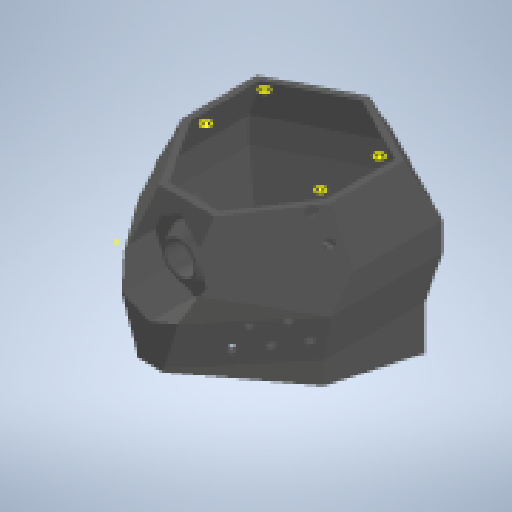
# Autodesk Inventor part: head_bace
Saved by Autodesk Inventor 2026.1 (Build 301233020, 233B)
## iProperties
Created: 2024-02-25
Part Number: head_bace
Material: 一般
Document SubType Name: Modeling
Designer: hibik
Density: 1 g/cm^3
Appearance: 既定
Author: hibik
Autodesk Inventor part; units mm, degrees
ref_plane "YZ Plane" through (0, 0, 0) normal (1, 0, 0) x (0, 1, 0)
ref_plane "XZ Plane" through (0, 0, 0) normal (0, 1, 0) x (-1, 0, 0)
sketch "スケッチ1" plane through (0, 0, 0) normal (0, 1, 0) x (-1, 0, 0)
  line L0 (-17.5, -21) -> (0, 0)
  line L1 (0, 0) -> (17.5, -21)
  line L2 (17.5, -21) -> (17.5, -41)
  line L3 (17.5, -41) -> (0, -50)
  line L4 (0, -50) -> (-17.5, -41)
  line L5 (-17.5, -41) -> (-17.5, -21)
  line L6 (0, -60) -> (0, 10) projected
  line L7 (24.5, 0) -> (-24.5, 0) projected
  dimension "d0" = 50
  dimension "d12" = 35
  dimension "d13" = 20
  dimension "d14" = 21
  constraints: 12 end point, 2 horizontal alignment, 1 coincident, 1 point on line, 1 vertical, 2 other
  measures "d0" distance of L0.end L3.end
  measures "d12" distance between parallel lines of L5 L2
  measures "d13" distance of L4.end L0.start
  measures "d14" vertical distance of L0.end L1.end
extrude "押し出し1" add sketch "スケッチ1" along normal blind 18
chamfer "面取り1" distance 5 distance2 10 6 edges at (8.75, 18, -10.5) (17.5, 18, -31) (8.75, 18, -45.5) (-8.75, 18, -45.5) (-17.5, 18, -31) (-8.75, 18, -10.5) measured on face at (8.3659, 18, -10.8201) measured on face at (-8.3659, 18, -10.8201) measured on face at (8.5213, 18, -45.0554) measured on face at (17, 18, -31) measured on face at (-17, 18, -31) measured on face at (-8.5213, 18, -45.0554)
extrude "押し出し2" add sketch "スケッチ1" against normal blind 5
ref_plane "作業平面1" through (0, 8, 0) normal (0, -0.7881104, 0.6155339) x (1, 0, 0)
sketch "スケッチ2" plane through (0, 8, 0) normal (0, -0.7881104, 0.6155339) x (1, 0, 0)
  line L0 (0, 0) -> (17.5, -16.5503) projected
  line L1 (-17.5, -16.5503) -> (0, 0) projected
  line L2 (-5, -4.7287) -> (-5, -4.7287)
  line L3 (-5, -4.7287) -> (5, -4.7287)
  line L4 (13.3346, -12.611) -> (5, -4.7287)
  line L5 (-5, -4.7287) -> (-23.6413, -26.9446)
  line L6 (5, -4.7287) -> (18.7173, -21.0763)
  line L7 (-23.6413, -26.9446) -> (-26.2109, -24.7885)
  line L8 (-26.2109, -24.7885) -> (-17.5, -16.5503)
  line L9 (17.5, -16.5503) -> (23.8178, -21.8516)
  line L10 (23.8178, -21.8516) -> (18.7173, -21.0763)
  point P0 (0, -4.9243)
  dimension "d9" = 10
  dimension "d25" = 130
  dimension "d26" = 130
  constraints: 18 end point, 4 point on line, 2 collinear, 1 horizontal, 1 parallel
  measures "d9" distance of L2.end L3.end
  measures "d25" angle of L3 L5
  measures "d26" angle of L6 L3
extrude "押し出し3" cut sketch "スケッチ2" against normal through all
chamfer "面取り2" distance 2 distance2 8 6 edges at (-8.75, -5, -10.5) (-17.5, -5, -31) (-8.75, -5, -45.5) (8.75, -5, -45.5) (17.5, -5, -31) (8.75, -5, -10.5) measured on face at (17, -5, -31) measured on face at (-8.5213, -5, -45.0554) measured on face at (8.3659, -5, -10.8201) measured on face at (-17, -5, -31) measured on face at (-8.3659, -5, -10.8201) measured on face at (8.5213, -5, -45.0554)
sketch "スケッチ3" plane through (0, -5, 0) normal (0, -1, 0) x (1, 0, 0)
  line L0 (0, -3.1241) -> (15.5, -21.7241) projected
  line L1 (-15.5, -21.7241) -> (0, -3.1241) projected
  line L2 (-15.5, -39.7796) -> (-15.5, -21.7241) projected
  line L3 (0, -47.751) -> (-15.5, -39.7796) projected
  line L4 (15.5, -39.7796) -> (0, -47.751) projected
  line L5 (15.5, -21.7241) -> (15.5, -39.7796) projected
  point P0 (0, 0)
extrude "押し出し4" add sketch "スケッチ3" along normal blind 8
ref_plane "作業平面2" through (0, -5, -3.1241) normal (0, -0.9770022, 0.2132292) x (-0.3818297, -0.1970734, -0.9029774)
sketch "スケッチ4" plane through (0, -5, -3.1241) normal (0, -0.9770022, 0.2132292) x (-0.3818297, -0.1970734, -0.9029774)
  line L0 (80, -28.4848) -> (-10, -28.4848)
  line L1 (-10, -28.4848) -> (-10, 40)
  line L2 (-10, 40) -> (80, 40)
  line L3 (80, 40) -> (80, -28.4848)
  point P0 (-3.8064, -1.5725)
  constraints: 8 end point, 2 parallel, 1 horizontal, 1 perpendicular
extrude "押し出し5" cut sketch "スケッチ4" along normal through all
ref_plane "作業平面3" through (-5, 8, -6) normal (0, 0, 1) x (1, 0, 0)
sketch "スケッチ5" plane through (-5, 8, -6) normal (0, 0, 1) x (1, 0, 0)
  line L0 (-30, 20) -> (40, 20)
  line L1 (40, 20) -> (40, -30)
  line L2 (40, -30) -> (-30, -30)
  line L3 (-30, -30) -> (-30, 20)
  point P0 (5, -8)
  constraints: 8 end point, 2 parallel, 1 horizontal, 1 perpendicular
extrude "押し出し6" cut sketch "スケッチ5" along normal through all
sketch "スケッチ6" plane through (-5, 8, -6) normal (0, 0, 1) x (1, 0, 0)
  line L0 (0, 0) -> (10, 0) projected
  circle A0 centre (5, 0) radius 5
  line L1 (9.9497, -4.9497) -> (5, -7)
  line L2 (5, -7) -> (0.0503, -4.9497)
  line L3 (0.0503, -4.9497) -> (-2, 0)
  line L4 (-2, 0) -> (0.0503, 4.9497)
  line L5 (0.0503, 4.9497) -> (5, 7)
  line L6 (5, 7) -> (9.9497, 4.9497)
  line L7 (9.9497, 4.9497) -> (12, 0)
  line L8 (12, 0) -> (9.9497, -4.9497)
  point P0 (5, -8)
  dimension "d29" = 7
  constraints: 16 end point, 2 midpoint, 1 coincident, 1 horizontal alignment, 1 vertical alignment, 19 other
  measures "d29" distance of point (5, 0) L5.end
extrude "押し出し7" cut sketch "スケッチ6" against normal blind 8 contours A0 L0 | L0 A0 | L1 L2 L3 L4 L5 L6 L7 L8
sketch "スケッチ8" plane through (-5, 8, -14) normal (0, 0, 1) x (1, 0, 0)
  line L0 (5, 0) -> (-12.5, 0) projected
  circle A0 centre (5, 0) radius 4
  line L1 (5, 4) -> (5, -4)
  line L2 (5, -5) -> (5, 0) projected
  point P0 (5, -8)
  dimension "d32" = 8
  constraints: 2 end point, 2 point on circle, 1 centre point, 1 midpoint, 1 point on line
  measures "d32" diameter of A0
revolve "回転1" add sketch "スケッチ8" angle 360 about axis through (0, 12, -14) along (0, -1, 0) contours L1 A0
sketch "スケッチ9" plane through (-15.5, -5, -21.7241) normal (-0.7452841, -0.2425356, 0.6210701) x (0.6214323, 0.0848617, 0.7788584)
  circle A0 centre (10.2962, 6.6564) radius 0.8
  circle A1 centre (12.0048, 1.9574) radius 0.8
  circle A2 centre (7.081, 2.8272) radius 0.8
  circle A3 centre (2.1573, 3.697) radius 0.8
  circle A4 centre (5.3724, 7.5262) radius 0.8
  line L0 (2.1573, 3.697) -> (7.081, 2.8272) construction
  line L1 (7.081, 2.8272) -> (12.0048, 1.9574) construction
  line L2 (12.0048, 1.9574) -> (7.081, 2.8272)
  line L3 (5.3724, 7.5262) -> (10.2962, 6.6564) construction
  line L4 (10.2962, 6.6564) -> (9.5429, 2.3923) construction
  line L5 (5.3724, 7.5262) -> (4.6191, 3.2621) construction
  line L6 (10.2962, 6.6564) -> (12.0048, 1.9574) construction
  line L7 (12.0048, 1.9574) -> (11.7379, 0.4469) construction
  line L8 (12.0048, 1.9574) -> (13.2927, 2.4257) construction
  line L9 (20.3897, -1.7904) -> (19.4508, 6.57) projected
  line L10 (0, 0) -> (20.3897, -1.7904) projected
  point P0 (26.9765, 2.9875)
  dimension "d34" = 1.6
  dimension "d35" = 5
  dimension "d36" = 5
  dimension "d37" = 7.9143
  dimension "d38" = 3
  constraints: 18 end point, 5 centre point, 4 equal radius, 4 perpendicular, 3 equal length, 2 midpoint, 1 collinear
  measures "d34" diameter of A1
  measures "d35" distance from line of L0.end L7
  measures "d36" distance from line of L3.end L8
  measures "d37" distance from line of L9 L1.end
  measures "d38" distance from line of L10 L1.end
sketch "スケッチ10" plane through (-12.5, 18, -25.1515) normal (-0.7660444, 0.3956576, 0.5065876) x (0.5515991, 0, 0.8341093)
  circle A0 centre (2.1738, -2.388) radius 0.8 projected
  circle A1 centre (0.2082, -6.8935) radius 0.8 projected
  point P0 (27.8741, -17.8951)
sketch "スケッチ11" plane through (0, -5, -3.1241) normal (0, -0.9770022, 0.2132292) x (0.9242327, -0.0814172, -0.3730484)
  line L0 (3.339, -1.8055) -> (-1.091, -3.6357) projected
  line L1 (-7.0564, -23.5137) -> (-1.091, -3.6357) projected
  line L2 (0, -40.594) -> (-7.0564, -23.5137) projected
  line L3 (28.6512, -28.7573) -> (0, -40.594) projected
  line L4 (21.5948, -11.677) -> (28.6512, -28.7573) projected
  line L5 (3.339, -1.8055) -> (21.5948, -11.677) projected
  line L6 (0, -40.594) -> (21.5948, -11.677)
  line L7 (-7.0564, -23.5137) -> (28.6512, -28.7573)
  circle A0 centre (10.7974, -26.1355) radius 4.25
  point P0 (-1.5725, 3.8064)
  dimension "d43" = 8.5
  constraints: 4 end point, 1 centre point, 1 midpoint
  measures "d43" diameter of A0
ref_plane "作業平面4" through (0, -10.0527, -30.9651) normal (0, -0.9770022, 0.2132292) x (1, 0, 0)
sketch "スケッチ12" plane through (0, -10.0527, -30.9651) normal (0, -0.9770022, 0.2132292) x (1, 0, 0)
  circle A0 centre (0, 0) radius 4.25 projected
  circle A1 centre (0, 0) radius 0.8
  point P0 (0, 32.3965)
  dimension "d46" = 1.6
  constraints: 1 centre point, 1 coincident
  measures "d46" diameter of A1
sketch "スケッチ13" plane through (0, 18, 0) normal (0, 1, 0) x (1, 0, 0)
  line L0 (-30, 50) -> (40, 50)
  line L1 (40, 50) -> (40, 0)
  line L2 (40, 0) -> (-30, 0)
  line L3 (-30, 0) -> (-30, 50)
  point P0 (0, 0)
  constraints: 8 end point, 2 parallel, 1 horizontal, 1 perpendicular
extrude "押し出し12" cut sketch "スケッチ13" against normal blind 1.5
sketch "スケッチ14" plane through (0, -5, -3.1241) normal (0, -0.9770022, 0.2132292) x (0.9242327, -0.0814172, -0.3730484)
  circle A0 centre (10.7974, -26.1355) radius 0.8 projected
  circle A1 centre (10.7974, -26.1355) radius 6 construction
  circle A2 centre (8.5064, -20.5901) radius 0.8
  line L0 (3.339, -1.8055) -> (-1.091, -3.6357) projected
  line L1 (1.124, -2.7206) -> (10.7974, -26.1355) construction
  circle A3 centre (5.2563, -23.8343) radius 0.8
  circle A4 centre (5.252, -28.4265) radius 0.8
  circle A5 centre (8.4962, -31.6767) radius 0.8
  circle A6 centre (13.0884, -31.6809) radius 0.8
  circle A7 centre (16.3386, -28.4367) radius 0.8
  circle A8 centre (16.3428, -23.8445) radius 0.8
  circle A9 centre (13.0986, -20.5944) radius 0.8
  circle A10 centre (10.7974, -26.1355) radius 8.5
  point P0 (-1.5725, 3.8064)
  dimension "d51" = 12
  dimension "d52" = 1.6
  dimension "d55" = 360
  dimension "d57" = 2.5
  constraints: 9 centre point, 2 coincident, 2 end point, 1 midpoint, 1 perpendicular, 1 point on line, 20 other
  measures "d52" diameter of A2
sketch "スケッチ15" plane through (-5, 8, -14) normal (0, 0, 1) x (1, 0, 0)
  circle A0 centre (5, 0) radius 4 projected
  point P0 (5, -8)
extrude "押し出し15" cut sketch "スケッチ15" along normal through all
shell "シェル1" thickness 1 removed faces 1 at (0, 16.5, -31.8164)
extrude "押し出し16" cut sketch "スケッチ9" against normal blind 3
extrude "押し出し17" cut sketch "スケッチ10" against normal blind 3
extrude "押し出し18" cut sketch "スケッチ14" against normal blind 3 contours A0 | A2 | A3 | A4 | A5 | A6 | A7 | A8 | A9
sketch "スケッチ16" plane through (0, -5, -3.1241) normal (0, -0.9770022, 0.2132292) x (0.9242327, -0.0814172, -0.3730484)
  circle A0 centre (5.027, -12.1681) radius 8.3124
  line L0 (-7.0564, -23.5137) -> (-1.091, -3.6357) projected
  line L1 (3.339, -1.8055) -> (21.5948, -11.677) projected
  circle A1 centre (8.5064, -20.5901) radius 0.8 projected
  circle A2 centre (5.027, -12.1681) radius 5.8124
  point P0 (-1.5725, 3.8064)
  dimension "d71" = 2.5
  constraints: 3 tangent, 2 centre point, 1 coincident
  measures "d71" radial gap between concentric circles of A0 A2
extrude "押し出し19" cut sketch "スケッチ16" against normal blind 3 contours A2
sketch "スケッチ17" plane through (-13.1038, -12, -39.8874) normal (0, 0.9770022, -0.2132292) x (1, 0, 0)
  line L0 (7.3538, -0.6324) -> (18.8538, -0.6324)
  line L1 (18.8538, -0.6324) -> (18.8538, -19.1324)
  line L2 (18.8538, -19.1324) -> (7.3538, -19.1324)
  line L3 (7.3538, -19.1324) -> (7.3538, -0.6324)
  circle A0 centre (13.1038, -9.1324) radius 0.8 projected
  line L4 (9.6038, -0.6324) -> (16.6038, -0.6324)
  line L5 (16.6038, -0.6324) -> (16.6038, -19.1324)
  line L6 (16.6038, -19.1324) -> (9.6038, -19.1324)
  line L7 (9.6038, -19.1324) -> (9.6038, -0.6324)
  point P0 (13.1038, -41.5289)
  point P1 (13.1038, -19.1324)
  point P2 (13.1038, -0.6324)
  point P3 (16.6038, -0.6324)
  dimension "d74" = 11.5
  dimension "d75" = 18.5
  dimension "d76" = 10
  dimension "d77" = 7
  constraints: 16 end point, 4 parallel, 3 midpoint, 2 horizontal, 2 perpendicular, 2 point on line, 1 vertical alignment
  measures "d74" distance of L1.end L2.end
  measures "d75" distance of L0.end L1.end
  measures "d76" distance from line of L2 A0.centre
  measures "d77" distance between parallel lines of L5 L7
extrude "押し出し20" add sketch "スケッチ17" along normal blind 3 contours L0 L7 L2 L3 | L0 L1 L2 L5
sketch "スケッチ18" plane through (-13.1038, -9.069, -40.5271) normal (0, 0.9770022, -0.2132292) x (1, 0, 0)
  line L0 (6.3538, 0.3676) -> (19.8538, 0.3676)
  line L1 (19.8538, 0.3676) -> (19.8538, -20.1324)
  line L2 (19.8538, -20.1324) -> (6.3538, -20.1324)
  line L3 (6.3538, -20.1324) -> (6.3538, 0.3676)
  line L4 (9.6038, -0.6324) -> (7.3538, -0.6324) projected
  line L5 (7.3538, -0.6324) -> (7.3538, -19.1324) projected
  line L6 (7.3538, -19.1324) -> (9.6038, -19.1324) projected
  line L7 (18.8538, -19.1324) -> (18.8538, -0.6324) projected
  line L8 (16.6038, -19.1324) -> (18.8538, -19.1324) projected
  line L9 (9.6038, -19.1324) -> (16.6038, -19.1324)
  line L10 (9.6038, -0.6324) -> (18.8538, -0.6324)
  point P0 (13.1038, -41.5289)
  point P1 (7.3538, -0.6324)
  dimension "d80" = 1
  dimension "d81" = 1
  dimension "d82" = 1
  dimension "d85" = 1
  constraints: 10 end point, 2 horizontal, 1 collinear, 1 parallel, 1 vertical, 3 other
  measures "d80" distance between parallel lines of L3 L5
  measures "d81" distance between parallel lines of L1 L7
  measures "d82" distance between parallel lines of L6 L2
extrude "押し出し21" add sketch "スケッチ18" against normal up to surface (3 mm away)
extrude "押し出し22" add sketch "スケッチ18" along normal blind 3
sketch "スケッチ19" plane through (-5, 8, -14) normal (0, 0, 1) x (1, 0, 0)
  circle A0 centre (5, 0) radius 2.5
  point P0 (5, -8)
  point P1 (12, 0)
  point P2 (5, 7)
  dimension "d88" = 5
  constraints: 1 centre point, 1 horizontal alignment, 1 vertical alignment
  measures "d88" diameter of A0
extrude "押し出し23" cut sketch "スケッチ19" against normal blind 3
sketch "スケッチ20" plane through (-5, 8, -14) normal (0, 0, 1) x (1, 0, 0)
  circle A0 centre (5, 0) radius 2.5 projected
  circle A1 centre (5, 0) radius 4.5
  point P0 (5, -8)
  dimension "d91" = 9
  constraints: 1 centre point, 1 coincident
  measures "d91" diameter of A1
extrude "押し出し24" add sketch "スケッチ20" along normal blind 4
sketch "スケッチ21" plane through (8.0824, 8, -15) normal (0, 0, -1) x (-0.9238795, -0.3826834, 0)
  circle A0 centre (7.4672, 3.093) radius 2.5 projected
  circle A1 centre (7.4672, 3.093) radius 4.5 projected
  circle A2 centre (7.4672, 3.093) radius 3
  point P0 (10.5286, -4.298)
  dimension "d94" = 6
  constraints: 1 centre point, 1 coincident
  measures "d94" diameter of A2
extrude "押し出し25" cut sketch "スケッチ21" against normal blind 1 contours A2
chamfer "面取り3" distance 2 distance2 4 1 edges at (-4.5, 8, -10) measured on face at (-4, 8, -10)
fillet "フィレット1" radius 0.4 2 edges at (-2.5001, 8, -10) (-2.5, 8, -10)
mirror "ミラー2" about plane through (0, 0, 0) normal (1, 0, 0) of "押し出し16", "押し出し17"
sketch "スケッチ22" plane through (0, 16.5, 0) normal (0, 1, 0) x (1, 0, 0)
  circle A0 centre (-10.2746, 36.8098) radius 0.8 projected
  circle A1 centre (-10.2746, 26.2907) radius 0.8 projected
  circle A2 centre (-10.2746, 26.2907) radius 2.5
  circle A3 centre (-10.2746, 36.8098) radius 2.5
  point P0 (0, 0)
  dimension "d101" = 5
  dimension "d102" = 5
  constraints: 2 centre point, 2 coincident
  measures "d101" diameter of A2
  measures "d102" diameter of A3
ref_plane "作業平面5" through (0, 13.5, 0) normal (0, 1, 0) x (1, 0, 0)
sketch "スケッチ23" plane through (0, 13.5, 0) normal (0, 1, 0) x (1, 0, 0)
  line L0 (0, 45.6504) -> (-13.632, 38.6397) projected
  line L1 (-13.632, 38.6397) -> (-13.632, 25.3226) projected
  line L2 (-13.632, 25.3226) -> (-5.8042, 13.4857) projected
  line L3 (-5.8042, 13.4857) -> (-5.8042, 15) projected
  line L4 (-5.8042, 15) -> (5.8042, 15) projected
  line L5 (5.8042, 15) -> (5.8042, 13.4857) projected
  line L6 (5.8042, 13.4857) -> (13.632, 25.3226) projected
  line L7 (13.632, 25.3226) -> (13.632, 38.6397) projected
  line L8 (13.632, 38.6397) -> (0, 45.6504) projected
  line L9 (-3.6213, 14) -> (-3.6213, 10.2956) projected
  line L10 (-3.6213, 10.2956) -> (-5, 10.2956) projected
  line L11 (-5, 10.2956) -> (-14.75, 25.0393) projected
  line L12 (-14.75, 25.0393) -> (-14.75, 39.3219) projected
  line L13 (-14.75, 39.3219) -> (0, 46.9076) projected
  line L14 (0, 46.9076) -> (14.75, 39.3219) projected
  line L15 (14.75, 39.3219) -> (14.75, 25.0393) projected
  line L16 (14.75, 25.0393) -> (5, 10.2956) projected
  line L17 (5, 10.2956) -> (3.6213, 10.2956) projected
  line L18 (3.6213, 10.2956) -> (3.6213, 14) projected
  line L19 (3.6213, 14) -> (-3.6213, 14) projected
  point P0 (0, 0)
sketch "スケッチ24" plane through (0, 13.5, 0) normal (0, 1, 0) x (1, 0, 0)
  circle A0 centre (-10.2746, 36.8098) radius 2.5 construction
  circle A1 centre (-10.2746, 26.2907) radius 2.5 construction
  circle A2 centre (-10.2746, 36.8098) radius 0.8 projected
  circle A3 centre (-10.2746, 26.2907) radius 0.8 projected
  line L0 (-13.632, 38.6397) -> (-13.632, 25.3226) construction
  line L1 (0, 45.6504) -> (-13.632, 38.6397) construction
  line L2 (-13.632, 25.3226) -> (-5.8042, 13.4857) construction
  line L3 (-13.632, 34.3098) -> (-10.2746, 34.3098)
  line L4 (-8.0514, 37.9532) -> (-9.4979, 40.7658)
  line L5 (-13.632, 28.7907) -> (-10.2746, 28.7907)
  line L6 (-8.8956, 24.2054) -> (-11.6769, 22.3661)
  line L7 (-13.632, 38.6397) -> (-13.632, 34.3098)
  line L8 (-9.4979, 40.7658) -> (-13.632, 38.6397)
  arc A4 (-10.2746, 34.3098) -> (-8.0514, 37.9532) centre (-10.2746, 36.8098) ccw
  arc A5 (-8.8956, 24.2054) -> (-10.2746, 28.7907) centre (-10.2746, 26.2907) ccw
  line L9 (-13.632, 28.7907) -> (-13.632, 25.3226)
  line L10 (-13.632, 25.3226) -> (-11.6769, 22.3661)
  point P0 (0, 0)
  constraints: 16 end point, 8 point on circle, 8 tangent, 4 perpendicular, 4 point on line, 2 centre point, 2 collinear, 1 vertical
sketch "スケッチ27" plane through (0, 16.5, 0) normal (0, 1, 0) x (1, 0, 0)
  circle A0 centre (-10.2746, 36.8098) radius 0.8 construction
  line L0 (-12.132, 37.7244) -> (0, 43.9637) construction
  line L1 (-12.132, 25.3974) -> (-12.132, 37.7244) construction
  arc A1 (-10.2746, 34.3098) -> (-8.0514, 37.9532) centre (-10.2746, 36.8098) ccw
  line L2 (-8.0514, 37.9532) -> (-8.8119, 39.4318)
  line L3 (-10.2746, 34.3098) -> (-12.132, 34.3098)
  line L4 (-12.132, 34.3098) -> (-12.132, 37.7244)
  line L5 (-12.132, 37.7244) -> (-8.8119, 39.4318)
  line L6 (-12.132, 34.3098) -> (-12.132, 37.7244)
  point P0 (0, 0)
  point P1 (-12.132, 28.7907)
  dimension "d113" = 2.5
  constraints: 10 end point, 2 collinear, 2 perpendicular, 2 point on circle, 2 point on line, 2 tangent, 1 centre point, 1 coincident
  measures "d113" radius of A1
sketch "スケッチ28" plane through (0, 13.5, 0) normal (0, 1, 0) x (1, 0, 0)
  line L0 (-13.632, 34.3098) -> (-10.2746, 34.3098) projected
  line L1 (-13.632, 38.6397) -> (-13.632, 34.3098) projected
  line L2 (-9.4979, 40.7658) -> (-13.632, 38.6397) projected
  line L3 (-8.0514, 37.9532) -> (-9.4979, 40.7658) projected
  circle A0 centre (-10.2746, 36.8098) radius 2.5 construction
  arc A1 (-10.2746, 34.3098) -> (-8.0514, 37.9532) centre (-10.2746, 36.8098) ccw projected
  point P0 (0, 0)
loft "ロフト2" add profiles "スケッチ27", "スケッチ28"
extrude "押し出し27" cut sketch "スケッチ22" against normal blind 3 contours A0
mirror "ミラー3" about plane through (0, 0, 0) normal (1, 0, 0) of "ロフト2", "押し出し27"
equation "\"d85\" = d80"
